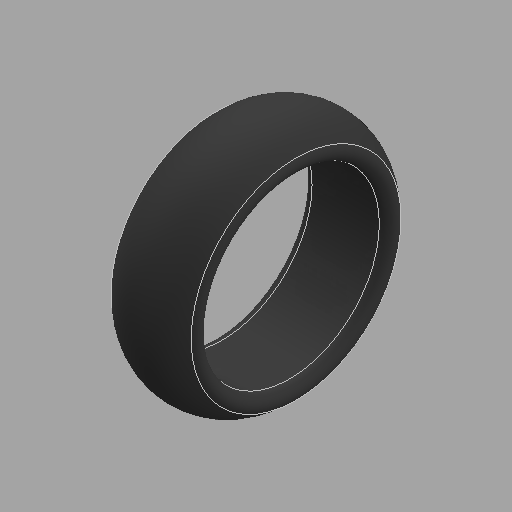
# Autodesk Inventor part: tire
Saved by Autodesk Inventor 2024 (Build 280153000, 153)
## iProperties
Created: 2024-04-09
Part Number: tire
Material: Rubber
Document SubType Name: Modeling
Designer: Alex
Density: 0.93 g/cm^3
Appearance: Rubber - Black
Author: Alex
Autodesk Inventor part; units mm, degrees
ref_plane "YZ Plane" through (0, 0, 0) normal (1, 0, 0) x (0, 1, 0)
sketch "Sketch1" plane through (0, 0, 0) normal (0, 1, 0) x (-1, 0, 0)
  line L0 (0, 0) -> (0, -40) construction
  line L1 (-15, -40) -> (15, -40)
  line L2 (0, -40) -> (0, -49.0309) construction
  arc A0 (17.8571, -46.7994) -> (15, -40) centre (15, -44) ccw
  arc A1 (-17.8571, -46.7994) -> (17.8571, -46.7994) centre (0, -29.3031) ccw
  arc A2 (-15, -40) -> (-17.8571, -46.7994) centre (-15, -44) ccw
  line L3 (17.8571, -46.7994) -> (-17.8571, -46.7994) construction
  line L4 (15, -40) -> (-15, -40) construction
  line L5 (28.1627, 0) -> (-28.1627, 0) projected
  line L6 (17.8571, 0) -> (-17.8571, 0)
  point P0 (0, -54.3031)
  dimension "d1" = 30
  dimension "d5" = 4
  dimension "d6" = 80
  dimension "d7" = 25
  constraints: 12 end point, 8 point on circle, 3 centre point, 3 point on line, 2 tangent, 2 vertical, 2 vertical alignment, 1 collinear, 1 equal radius, 1 horizontal, 1 midpoint, 1 perpendicular
  measures "d1" distance of L1.start L1.end
  measures "d5" radius of A2
  measures "d6" diameter of L1 L5
  measures "d7" radius of A1
revolve "Revolution1" add sketch "Sketch1" angle 360 about axis through (-10, 0, 0) along (1, 0, 0)
ref_plane "Work Plane3" through (0, 0, 0) normal (1, 0, 0) x (0, 1, 0)
ref_plane "Work Plane1" through (15, 0, 0) normal (1, 0, 0) x (0, 1, 0)
ref_plane "Work Plane2" through (-15, 0, 0) normal (1, 0, 0) x (0, 1, 0)
ref_plane "Work Plane5" through (0, 0, 0) normal (1, 0, 0) x (0, 1, 0)
body "Solid1"
